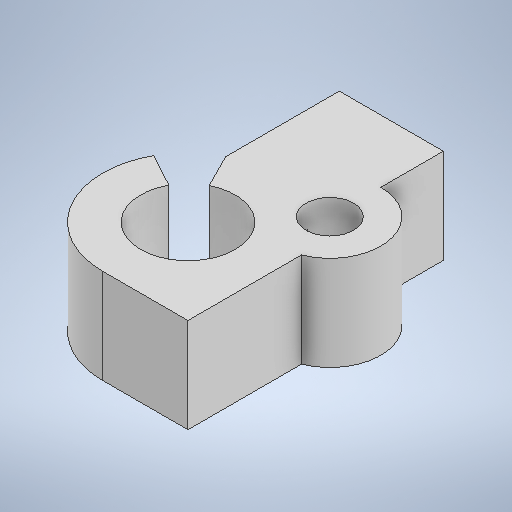
# Autodesk Inventor part: ikatire_rod3.0
Saved by Autodesk Inventor 2025 (Build 290162000, 162)
## iProperties
Created: 2024-07-11
Part Number: ikatire_rod3.0
Material: 一般
Document SubType Name: Modeling
Designer: Saigusa
Density: 1 g/cm^3
Appearance: 既定
Author: Saigusa
Autodesk Inventor part; units mm, degrees
ref_plane "YZ Plane" through (0, 0, 0) normal (1, 0, 0) x (0, 1, 0)
ref_plane "XZ Plane" through (0, 0, 0) normal (0, 1, 0) x (-1, 0, 0)
ref_plane "XY Plane" through (0, 0, 0) normal (0, 0, 1) x (1, 0, 0)
sketch "スケッチ1" plane through (0, 0, 0) normal (0, 1, 0) x (-1, 0, 0)
  circle A0 centre (0, 0) radius 1.25
  line L0 (0, 0) -> (0, 8.5)
  line L1 (0, 8.5) -> (50, 8.5)
  line L2 (50, 8.5) -> (-50, 8.5)
  line L3 (0, 0) -> (-4, 0)
  line L4 (-4, 0) -> (-4, 8.5)
  line L5 (-4, 8.5) -> (-4, 2.5)
  line L6 (-4, 2.5) -> (-1, 2.5)
  line L7 (-1, 2.5) -> (-1, 8.5)
  circle A1 centre (0, 0) radius 2.6926
  line L8 (-1, 8.5) -> (3.5, 8.5)
  line L9 (3.5, 8.5) -> (3.5, 4)
  line L10 (3.5, 4) -> (-1, 4)
  line L11 (-1, 4) -> (-1, 8.5)
  circle A2 centre (3.5, 4) radius 4.5
  circle A3 centre (3.5, 4) radius 2.5
  line L12 (0, 0) -> (5.5, 0)
  line L13 (5.5, 0) -> (5.5, -6)
  line L14 (5.5, -6) -> (0, -6)
  line L15 (0, -6) -> (0, 0)
  line L16 (5.5, 0) -> (3.5, 4)
  line L17 (3.5, 4) -> (7.4571, 1.8573)
  line L18 (-2.6926, 0) -> (0, 0)
  line L19 (0, 0) -> (0, -6)
  line L20 (0, -6) -> (-2.6926, -6)
  line L21 (-2.6926, -6) -> (-2.6926, 0)
  point P0 (0, -2.6926)
  point P1 (4.618, 1.7639)
  point P2 (5.6984, 2.8096)
  point P3 (0, 1.25)
  point P4 (-0.0608, 1.2485)
  point P5 (0, 1.1716)
  dimension "d0" = 2.5
  dimension "d1" = 8.5
  dimension "d2" = 50
  dimension "d3" = 100
  dimension "d4" = 4
  dimension "d5" = 6
  dimension "d6" = 3
  dimension "d7" = 4.5
  dimension "d8" = 4.5
  dimension "d9" = 5
  dimension "d10" = 5.5
  dimension "d11" = 6
  dimension "d12" = 35
  constraints: 44 end point, 6 horizontal, 6 parallel, 5 perpendicular, 4 centre point, 4 coincident, 4 point on circle, 4 point on line, 1 vertical
  measures "d0" diameter of A0
  measures "d1" distance of L0.start L0.end
  measures "d2" distance of L0.end L1.end
  measures "d3" distance of L1.end L2.end
  measures "d4" distance of L0.start L3.end
  measures "d5" distance of L4.end L5.end
  measures "d6" distance of L5.end L6.end
  measures "d7" distance of L9.end L10.end
  measures "d8" distance of L8.end L9.end
  measures "d9" diameter of A3
  measures "d10" distance of L13.end L14.end
  measures "d11" distance of L12.end L13.end
  measures "d12" angle of L16 L17
extrude "押し出し1" add sketch "スケッチ1" along normal blind 5 contours L12 A2 A1 L15 A0 | A0 A2 L12 | A0 L0 A1 L12 A2 | L15 A1 L3 A0 | L12 A1 A2 | L0 A2 A0 | A0 A2 A1 L0 | L3 A1 A2 A0 | A1 A2 L13 L14 L15 | A1 L12 L13 A2 | A1 L0 L10 A3 L16 L12 | A1 A2 L10 L0 | A1 L7 A2 | L10 A2 L0 | L0 A2 L9 A3 L10 | L17 A3 L9 A2 | L7 L2 L0 A2 | L0 L1 A2 picked at (-0.0068, 1.2062)
sketch "スケッチ2" plane through (0, 0, -6) normal (0, 0, -1) x (-1, 0, 0)
  line L0 (5.5, 0) -> (5.5, 5) projected
  line L1 (5.5, 0) -> (3, 0)
  line L2 (3, 0) -> (3, 2.5)
  line L3 (3, 2.5) -> (5.5, 2.5)
  line L4 (5.5, 2.5) -> (5.5, 0)
  circle A0 centre (3, 2.5) radius 1.6
  point P0 (0, 0)
  dimension "d15" = 2.5
  dimension "d16" = 2.5
  dimension "d17" = 3.2
  constraints: 8 end point, 2 parallel, 1 centre point, 1 coincident, 1 horizontal, 1 perpendicular
  measures "d15" distance of L2.end L3.end
  measures "d16" distance of L1.end L2.end
  measures "d17" diameter of A0
extrude "押し出し2" cut sketch "スケッチ2" against normal blind 6 contours A0 L2 L3 | L3 L2 A0
